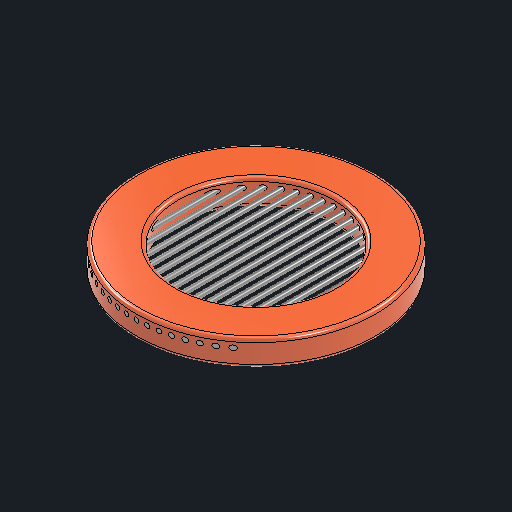
# Autodesk Inventor part: mesh
Saved by Autodesk Inventor 2026 (Build 300175050, 175E)
## iProperties
Created: 2025-08-28
Part Number: mesh
Material: Stainless Steel
Document SubType Name: Modeling
Designer: queezz
Density: 8 g/cm^3
Appearance: Semi-Polished
Author: queezz
Autodesk Inventor part; units mm, degrees
ref_plane "YZ Plane" through (0, 0, 0) normal (1, 0, 0) x (0, 1, 0)
ref_plane "XZ Plane" through (0, 0, 0) normal (0, 1, 0) x (-1, 0, 0)
ref_plane "XY Plane" through (0, 0, 0) normal (0, 0, 1) x (1, 0, 0)
sketch "Sketch1" plane through (0, 0, 0) normal (0, 0, 1) x (1, 0, 0)
  circle A0 centre (0, 0) radius 0.275
  dimension "d0" = 0.55
  constraints: 1 centre point, 1 coincident
  measures "d0" diameter of A0
extrude "Extrusion1" add sketch "Sketch1" along normal mid plane 30
pattern_linear "Rectangular Pattern1" count 15 spacing 1.2 along (1, 0, 0) of "Extrusion1" first direction both ways yes
sketch "Sketch3" plane through (0, 0, 0) normal (0, 1, 0) x (-1, 0, 0)
  line L0 (0.275, -15) -> (0.275, 15) projected
  circle A0 centre (0, 0) radius 13.9
  circle A1 centre (0, 0) radius 20
  dimension "d17" = 27.8
  dimension "d18" = 40
  constraints: 2 centre point, 2 coincident
  measures "d17" diameter of A0
  measures "d18" diameter of A1
extrude "Extrusion3" cut sketch "Sketch3" along normal through all both and the other way through all
sketch "Sketch2" plane through (0, 0, 0) normal (0, 1, 0) x (-1, 0, 0)
  circle A0 centre (0, 0) radius 13.9
  circle A1 centre (0, 0) radius 9.05
  dimension "d6" = 27.8
  dimension "d7" = 18.1
  constraints: 2 centre point, 2 coincident
  measures "d6" diameter of A0
  measures "d7" diameter of A1
extrude "Extrusion2" add sketch "Sketch2" along normal blind 1 and the other way blind 2 separate body
combine bodies "Combine1" operation type subtract main body 2 bodies to subtract 1 keep tools yes
fillet "Fillet1" radius 0.4 4 edges at (9.05, 1, 0) (13.9, 1, 0) (13.9, -2, 0) (9.05, -2, 0)
equation "\"d0\" = wire"
equation "\"wire\" = 0.55"
